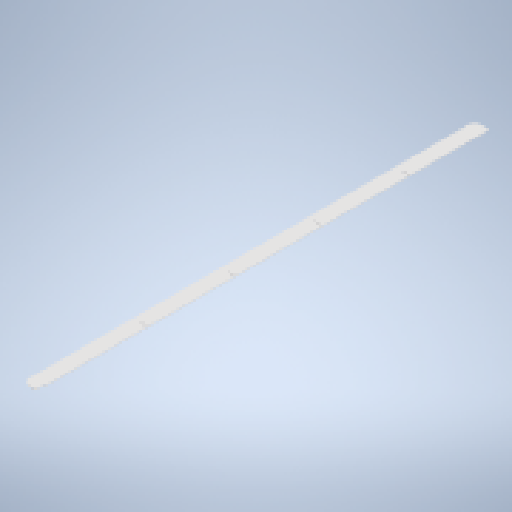
# Autodesk Inventor part: BSH 023 rib butt end
Saved by Autodesk Inventor 2025 (Build 290162010, 162A)
## iProperties
Created: 2024-07-31
Part Number: BSH 023 rib butt end
Material: Steel
Document SubType Name: Sheet Metal
Designer: pokla
Density: 7.85 g/cm^3
Sheet Metal Rule: AISI304 3mm Die 32
Appearance: Default
Stock Number: БШК 023 шпангоут торец
Author: pokla
Autodesk Inventor part; units mm, degrees
ref_plane "YZ Plane" through (0, 0, 0) normal (1, 0, 0) x (0, 1, 0)
ref_plane "XZ Plane" through (0, 0, 0) normal (0, 1, 0) x (-1, 0, 0)
ref_plane "XY Plane" through (0, 0, 0) normal (0, 0, 1) x (1, 0, 0)
sketch "Sketch1" plane through (0, 0, 0) normal (0, 0, 1) x (1, 0, 0)
  line L0 (-95, 2900.463) -> (0, 2900.463)
  line L1 (0, 2900.463) -> (0, 0)
  line L2 (0, 0) -> (-95, 0)
  line L3 (-95, 0) -> (-95, 2900.463)
  line L4 (-12, 53) -> (0, 53)
  line L5 (0, 53) -> (0, 0)
  line L6 (0, 0) -> (-12, 0)
  line L7 (-12, 0) -> (-12, 53)
  point P0 (-12, 0)
  dimension "d0" = 95
  dimension "d1" = 2900.463
  dimension "d10" = 12
  dimension "d11" = 53
  measures "d0" distance of L0.start L0.end
  measures "d1" distance of L2.end L0.start
  measures "d10" distance of L1.end L6.end
  measures "d11" distance of L1.end L4.end
extrude "Plate1" add sketch "Sketch1" along normal blind 3 contours L0 L1 L4 L7 L2 L3
sketch "Sketch2" plane through (0, 0, 3) normal (0, 0, 1) x (1, 0, 0)
  line L0 (0, 0) -> (0, 2900.463) projected
  line L1 (0, 2391.207) -> (-48.5, 2391.207)
  line L2 (-48.5, 2391.207) -> (-48.5, 2388.007)
  line L3 (-48.5, 2388.007) -> (0, 2388.007)
  line L4 (0, 2388.007) -> (0, 2391.207)
  point P0 (0, 2388.007)
  dimension "d3" = 509.256
  dimension "d4" = 3.2
  dimension "d5" = 48.5
  constraints: 8 end point, 2 parallel, 1 horizontal, 1 perpendicular, 1 point on line
  measures "d3" distance of L1.start L0.end
  measures "d4" distance between parallel lines of L3 L1
  measures "d5" distance of L1.start L1.end
extrude "Extrusion1" cut sketch "Sketch2" against normal through all
pattern_linear "Rectangular Pattern1" count 4 spacing 560 along (0, -1, 0) of "Extrusion1"
fillet "Corner Round1" radius 40 2 edges at (-95, 2900.463, 1.5) (-95, 0, 1.5)
equation "\"d2\" = Thickness"
equation "\"BendReliefWidth\" = Thickness"
equation "\"BendReliefDepth\" = 0.5 * Thickness"
equation "\"CornerReliefSize\" = 4 * Thickness"
equation "\"MinimumRemnant\" = 2 * Thickness"
equation "\"TransitionRadius\" = BendRadius"
equation "\"JacobiRadiusSize\" = BendRadius"
equation "\"GapSize\" = Thickness"
equation "\"Thickness\" = 3"
equation "\"BendRadius\" = 5"
body "Solid1"
